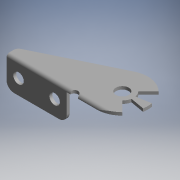
# Autodesk Inventor part: MHPUS306-Ab_fixed_right
Saved by Autodesk Inventor 2017.3 (Build 213256000, 256)
## iProperties
Part Number: MHPUS306-Ab_fixed_right
Material: Generic
Catalog Web Link: www.cadenas.de
Description: MHPUS_b_fixed_right-Cable Carriers Flap Open - Close Type
Vendor: MISUMI
Document SubType Name: Modeling
Designer: partserver
Manufacturer: MISUMI
Mass: 4.26369 g
Surface Area: 48.7004 cm^2
Volume: 4.26369 cm^3
Density: 1 g/cm^3
Appearance: PSOLRGB-192-192-192
Category: PARTsolutions
Company: MISUMI
Title: MHPUS306-Ab_fixed_right
Author: Cadenas PARTsolutions
Comments: Cable Carriers Flap Open - Close Type
PSOL_IDENT_0: {$CADENAS_DATA\23d-libs\misumi\metric\07_slide_rails\mhpus_bracket_fixed_right.prj},201 {VTYP=3D},{N
PSOL_IDENT_1: B=MHPUS306-Ab_fixed_right},{LINA=MHPUS306-Ab_fixed_right},{NN=MHPUS_b_fixed_right},{DATE=30.06.2021
PSOL_IDENT_2: 12:53:59},{GEOMDATE=28.08.2009 10:24:00},{VERSION=},{LINEID=80},{WBVAR=AD},{WBNUMERIC=}  {NB=MHPUS30
PSOL_IDENT_3: 6-Ab_fixed_right},{LINA=MHPUS306-Ab_fixed_right},{KT=DUMMY},{PN=MHPUS306-A},{NO=306},{MAT=Low Carbon
PSOL_IDENT_4: Steel},{ST=Trivalent Bright Chromate Plating},{AD=A},{ADALG= 'A', 'Outer circumference', 'B', 'Inne
PSOL_IDENT_5: r circumference' },{HH=34},{F=40},{T=24},{J=20},{N=7.0},{LL=60},{P1F=35.6},{P2F=55.6},{P1FX=32},{P2F
PSOL_IDENT_6: X=52},{R4=8.000},{R1=2.000},{R2=5.000},{R24=35.000},{R25=10.000},{R26=7.500},{END=1}
NB: MHPUS306-Ab_fixed_right
NN: MHPUS_b_fixed_right
NT: Cable Carriers Flap Open - Close Type
NBSYN: $PN.b_fixed_right
LINA: MHPUS306-Ab_fixed_right
CATALOG: Misumi
PN: MHPUS306-A
NO: 306
MAT: Low Carbon Steel
ST: Trivalent Bright Chromate Plating
AD: Outer circumference
HH: 34
F: 40
T: 24
J: 20
N: 7
LL: 60
P1F: 35.6
P2F: 55.6
P1FX: 32
P2FX: 52
R4: 8
R1: 2
R2: 5
R24: 35
R25: 10
R26: 7.5
SUPPLIER: MISUMI
ARTICLENO: MHPUS306-Ab_fixed_right
BOMINFO: MHPUS306-Ab_fixed_right
CREATOR: CADENAS GmbH
Autodesk Inventor part; units mm, degrees
sketch "Sketch_1" plane through (0, 0, 0) normal (0, 0, 1) x (1, 0, 0)
  arc A0 (-16.7417, 19.952) -> (-16.7417, 14.048) centre (0, 17) ccw
  line L0 (-16.7417, 14.048) -> (-7.3861, 15.6976)
  arc A1 (-7.3861, 15.6976) -> (-5.3033, 11.6967) centre (0, 17) ccw
  line L1 (-5.3033, 11.6967) -> (-12.0208, 4.9792)
  arc A2 (-12.0208, 4.9792) -> (0, 0) centre (0, 17) ccw
  line L2 (0, 0) -> (60, 0)
  line L3 (60, 0) -> (60, 4.67)
  arc A3 (60, 4.67) -> (58.0834, 7.7293) centre (56.6, 4.67) ccw
  line L4 (58.0834, 7.7293) -> (7.4171, 32.2966)
  arc A4 (7.4171, 32.2966) -> (-12.0208, 29.0208) centre (0, 17) ccw
  line L5 (-12.0208, 29.0208) -> (-5.3033, 22.3033)
  arc A5 (-5.3033, 22.3033) -> (-7.3861, 18.3024) centre (0, 17) ccw
  line L6 (-7.3861, 18.3024) -> (-16.7417, 19.952)
  circle A6 centre (0, 17) radius 4.25
  constraints: 14 end point, 12 point on circle, 7 centre point
extrude "Extrusion1" add sketch "Sketch_1" along normal blind 20
sketch "Sketch_2" plane through (0, 0, 0) normal (1, 0, 0) x (0, 1, 0)
  line L0 (39, 25) -> (-5, 25)
  line L1 (-5, 25) -> (-5, -5)
  line L2 (-5, -5) -> (39, -5)
  line L3 (39, -5) -> (39, 25)
  line L4 (2, 20) -> (0, 20)
  line L5 (0, 20) -> (0, 2)
  arc A0 (0, 2) -> (2, 0) centre (2, 2) ccw
  line L6 (2, 0) -> (34, 0)
  line L7 (34, 0) -> (34, 2)
  line L8 (34, 2) -> (3, 2)
  arc A1 (2, 3) -> (3, 2) centre (3, 3) ccw
  line L9 (2, 3) -> (2, 20)
  constraints: 20 end point, 4 point on circle, 2 centre point
extrude "Extrusion2" cut sketch "Sketch_2" along normal mid plane 120
sketch "Sketch_3" plane through (0, 0, 0) normal (0, 1, 0) x (-1, 0, 0)
  line L0 (22, 25) -> (-65, 25)
  line L1 (-65, 25) -> (-65, -5)
  line L2 (-65, -5) -> (22, -5)
  line L3 (22, -5) -> (22, 25)
  line L4 (17, 2) -> (-20, 2)
  line L5 (-20, 2) -> (-20, 15)
  arc A0 (-20, 15) -> (-25, 20) centre (-25, 15) ccw
  line L6 (-25, 20) -> (-55, 20)
  arc A1 (-55, 20) -> (-60, 15) centre (-55, 15) ccw
  line L7 (-60, 15) -> (-60, 0)
  line L8 (-60, 0) -> (17, 0)
  line L9 (17, 0) -> (17, 2)
  constraints: 20 end point, 4 point on circle, 2 centre point
extrude "Extrusion3" cut sketch "Sketch_3" along normal blind 34
sketch "Sketch4" plane through (20, 0, 2) normal (0, -1, 0) x (1, 0, 0)
  point P0 (8, 8)
hole "Hole1" at (28, 0, 10) direction (0, 1, 0) diameter 7 depth 2
sketch "Sketch5" plane through (20, 0, 2) normal (0, -1, 0) x (1, 0, 0)
  point P0 (32, 8)
hole "Hole2" at (52, 0, 10) direction (0, 1, 0) diameter 7 depth 2
sketch "Sketch_7" plane through (0, 0, 0) normal (0, 0, 1) x (1, 0, 0)
  circle A0 centre (15, 0) radius 2.5
  constraints: 1 centre point
extrude "Extrusion4" cut sketch "Sketch_7" along normal blind 20
ref_plane "fix_end_r_XY" through (0, 17, 0) normal (0, 0, 1) x (1, 0, 0)
ref_plane "fix_end_r_YZ" through (0, 17, 0) normal (1, 0, 0) x (0, 1, 0)
ref_plane "fix_end_r_ZX" through (0, 17, 0) normal (0, 1, 0) x (0, 0, 1)
ref_plane "free_end_r_XY" through (0, 17, 2) normal (0, 0, 1) x (1, 0, 0)
ref_plane "free_end_r_YZ" through (0, 17, 2) normal (1, 0, 0) x (0, 1, 0)
ref_plane "free_end_r_ZX" through (0, 17, 2) normal (0, 1, 0) x (0, 0, 1)
ref_plane "r_XY" through (0, 17, 26) normal (0, 0, 1) x (1, 0, 0)
ref_plane "r_YZ" through (0, 17, 26) normal (1, 0, 0) x (0, 1, 0)
ref_plane "r_ZX" through (0, 17, 26) normal (0, 1, 0) x (0, 0, 1)
body "Solid1"
